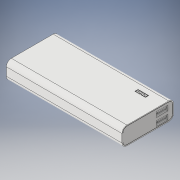
# Autodesk Inventor part: Battery
Saved by Autodesk Inventor 2018 (Build 220112000, 112)
## iProperties
Created: 2018-05-02
Part Number: Battery
Material: Generic
Document SubType Name: Modeling
Designer: Ajith Thomas
Density: 1 g/cm^3
Appearance: Default
Author: Ajith Thomas
Autodesk Inventor part; units mm, degrees
ref_plane "YZ Plane" through (0, 0, 0) normal (1, 0, 0) x (0, 1, 0)
ref_plane "XZ Plane" through (0, 0, 0) normal (0, 1, 0) x (-1, 0, 0)
ref_plane "XY Plane" through (0, 0, 0) normal (0, 0, 1) x (1, 0, 0)
sketch "Sketch1" plane through (0, 0, 0) normal (1, 0, 0) x (0, 1, 0)
  line L0 (11, 31.5) -> (-11, 31.5)
  line L1 (-11, 31.5) -> (-11, -31.5)
  line L2 (-11, -31.5) -> (11, -31.5)
  line L3 (11, -31.5) -> (11, 31.5)
  line L4 (11, 31.5) -> (-11, -31.5) construction
  line L5 (-11, 31.5) -> (11, -31.5) construction
  point P0 (0, 0)
  dimension "d0" = 22
  dimension "d1" = 63
  constraints: 12 end point, 2 midpoint, 2 parallel, 1 horizontal, 1 perpendicular
  measures "d0" distance of L2.end L1.end
  measures "d1" distance of L1.end L0.end
extrude "Extrusion1" add sketch "Sketch1" along normal mid plane 141
fillet "Fillet1" radius 6 4 edges at (0, 11, 31.5) (0, 11, -31.5) (0, -11, 31.5) (0, -11, -31.5)
sketch "Sketch2" plane through (70.5, 0, 0) normal (1, 0, 0) x (0, 0, -1)
  line L0 (10.5, 7) -> (24.5, 7)
  line L1 (24.5, 7) -> (24.5, 1)
  line L2 (24.5, 1) -> (10.5, 1)
  line L3 (10.5, 1) -> (10.5, 7)
  line L4 (31.5, -5) -> (31.5, 5) projected
  line L5 (25.5, 11) -> (-25.5, 11) projected
  line L6 (11.7, 5.85) -> (23.3, 5.85)
  line L7 (23.3, 5.85) -> (23.3, 4.6)
  line L8 (23.3, 4.6) -> (11.7, 4.6)
  line L9 (11.7, 4.6) -> (11.7, 5.85)
  line L10 (10.5, -2.5) -> (24.5, -2.5)
  line L11 (24.5, -2.5) -> (24.5, -8.5)
  line L12 (24.5, -8.5) -> (10.5, -8.5)
  line L13 (10.5, -8.5) -> (10.5, -2.5)
  line L14 (11.7, -3.65) -> (23.3, -3.65)
  line L15 (23.3, -3.65) -> (23.3, -4.9)
  line L16 (23.3, -4.9) -> (11.7, -4.9)
  line L17 (11.7, -4.9) -> (11.7, -3.65)
  point P0 (0, 0)
  dimension "d5" = 14
  dimension "d6" = 6
  dimension "d7" = 7
  dimension "d8" = 4
  dimension "d12" = 1.2
  dimension "d13" = 1.2
  dimension "d14" = 1.15
  dimension "d15" = 3.6
  dimension "d16" = 14
  dimension "d17" = 6
  dimension "d18" = 1.2
  dimension "d19" = 1.2
  dimension "d20" = 1.15
  dimension "d21" = 3.6
  dimension "d22" = 3.5
  constraints: 32 end point, 8 parallel, 4 horizontal, 4 perpendicular
  measures "d5" distance of L1.end L2.end
  measures "d6" distance of L0.end L1.end
  measures "d7" distance between parallel lines of L4 L1
  measures "d8" distance between parallel lines of L5 L0
  measures "d12" distance between parallel lines of L3 L9
  measures "d13" distance between parallel lines of L1 L7
  measures "d14" distance between parallel lines of L0 L6
  measures "d15" distance between parallel lines of L2 L8
  measures "d16" distance of L11.end L12.end
  measures "d17" distance of L10.end L11.end
  measures "d18" distance between parallel lines of L13 L17
  measures "d19" distance between parallel lines of L11 L15
  measures "d20" distance between parallel lines of L10 L14
  measures "d21" distance between parallel lines of L12 L16
  measures "d22" distance between parallel lines of L2 L10
extrude "Extrusion2" cut sketch "Sketch2" against normal blind 10
sketch "Sketch3" plane through (-70.5, 11, -25.5) normal (0, 1, 0) x (1, 0, 0)
  line L0 (110.1613, -6.5149) -> (123.1613, -6.5149)
  line L1 (123.1613, -6.5149) -> (123.1613, -10.5149)
  line L2 (123.1613, -10.5149) -> (110.1613, -10.5149)
  line L3 (110.1613, -10.5149) -> (110.1613, -6.5149)
  line L4 (110.6613, -7.0149) -> (112.6613, -7.0149)
  line L5 (112.6613, -7.0149) -> (112.6613, -10.0149)
  line L6 (112.6613, -10.0149) -> (110.6613, -10.0149)
  line L7 (110.6613, -10.0149) -> (110.6613, -7.0149)
  line L8 (115.9613, -10.0149) -> (113.9613, -10.0149)
  line L9 (113.9613, -10.0149) -> (113.9613, -7.0149)
  line L10 (113.9613, -7.0149) -> (115.9613, -7.0149)
  line L11 (115.9613, -7.0149) -> (115.9613, -10.0149)
  line L12 (119.2613, -10.0149) -> (117.2613, -10.0149)
  line L13 (117.2613, -10.0149) -> (117.2613, -7.0149)
  line L14 (117.2613, -7.0149) -> (119.2613, -7.0149)
  line L15 (119.2613, -7.0149) -> (119.2613, -10.0149)
  line L16 (122.5613, -10.0149) -> (120.5613, -10.0149)
  line L17 (120.5613, -10.0149) -> (120.5613, -7.0149)
  line L18 (120.5613, -7.0149) -> (122.5613, -7.0149)
  line L19 (122.5613, -7.0149) -> (122.5613, -10.0149)
  point P0 (70.5, -25.5)
  dimension "d25" = 13
  dimension "d26" = 4
  dimension "d27" = 2
  dimension "d28" = 3
  dimension "d29" = 0.5
  dimension "d30" = 0.5
  dimension "d33" = 3.3
  constraints: 40 end point, 4 parallel, 3 horizontal, 2 perpendicular, 24 other
  measures "d25" distance of L1.end L2.end
  measures "d26" distance of L0.end L1.end
  measures "d27" distance of L5.end L6.end
  measures "d28" distance of L4.end L5.end
  measures "d29" distance between parallel lines of L0 L4
  measures "d30" distance between parallel lines of L3 L7
  measures "d33" distance of L5.end L8.start
extrude "Extrusion3" cut sketch "Sketch3" against normal blind 0.25
sketch "Sketch4" plane through (70.5, -5, -31.5) normal (0, 0, -1) x (-1, 0, 0)
  line L0 (141, 10) -> (0, 10) construction
  line L1 (0, 0) -> (0, 10) construction
  line L2 (35, 5) -> (42, 5)
  line L3 (42, 5) -> (42, 8)
  line L4 (42, 8) -> (35, 8)
  line L5 (35, 8) -> (35, 5)
  line L6 (38.5, 5) -> (38.5, 8) construction
  line L7 (35, 6.5) -> (36.7876, 5)
  line L8 (35, 6.5) -> (37.3336, 6.5) construction
  line L9 (42, 6.5) -> (40.2124, 5)
  line L10 (42, 6.5) -> (42, 5)
  line L11 (40.2124, 5) -> (42, 5)
  point P0 (70.5, 5)
  dimension "d42" = 3
  dimension "d43" = 35
  dimension "d44" = 7
  dimension "d45" = 2
  dimension "d46" = 40
  constraints: 20 end point, 3 midpoint, 2 horizontal, 2 parallel, 2 perpendicular, 2 symmetric about line, 1 collinear, 1 equal length, 1 point on line
  measures "d42" distance of L3.end L2.end
  measures "d43" distance between parallel lines of L1 L5
  measures "d44" distance between parallel lines of L5 L3
  measures "d45" distance between parallel lines of L0 L4
  measures "d46" angle of L7 L8
extrude "Extrusion4" cut sketch "Sketch4" against normal blind 5 contours L7 L5 L4 L3 L9 L2
sketch "Sketch5" plane through (70.5, -5, -31.5) normal (0, 0, -1) x (-1, 0, 0)
  line L0 (0, 0) -> (0, 10) construction
  line L1 (0, 5) -> (141, 5) construction
  line L2 (141, 10) -> (141, 0) construction
  line L3 (13, 9) -> (27, 9)
  line L4 (27, 9) -> (27, 1)
  line L5 (27, 1) -> (13, 1)
  line L6 (13, 1) -> (13, 9)
  line L7 (13, 9) -> (27, 1) construction
  line L8 (27, 9) -> (13, 1) construction
  line L9 (26.75, 8.75) -> (13.25, 8.75)
  line L10 (13.25, 8.75) -> (13.25, 1.25)
  line L11 (13.25, 1.25) -> (26.75, 1.25)
  line L12 (26.75, 1.25) -> (26.75, 8.75)
  line L13 (35, 6.5) -> (35, 8) projected
  point P0 (70.5, 5)
  point P1 (20, 5)
  dimension "d49" = 14
  dimension "d50" = 8
  dimension "d51" = 0.25
  dimension "d52" = 8
  constraints: 22 end point, 4 midpoint, 4 parallel, 2 perpendicular, 1 horizontal, 1 point on line, 3 other
  measures "d49" distance of L4.end L5.end
  measures "d50" distance of L3.end L4.end
  measures "d51" distance between parallel lines of L3 L9
  measures "d52" distance between parallel lines of L13 L4
extrude "Extrusion5" cut sketch "Sketch5" against normal blind 0.1
sketch "Sketch6" plane through (70.5, 0, 0) normal (1, 0, 0) x (0, 0, -1)
  line L0 (10.5, 1) -> (10.5, 7) projected
  line L1 (10.5, 7) -> (24.5, 7) projected
  line L2 (24.5, 7) -> (24.5, 1) projected
  line L3 (24.5, 1) -> (10.5, 1) projected
  line L4 (10.5, -8.5) -> (10.5, -2.5) projected
  line L5 (10.5, -2.5) -> (24.5, -2.5) projected
  line L6 (24.5, -2.5) -> (24.5, -8.5) projected
  line L7 (24.5, -8.5) -> (10.5, -8.5) projected
  arc A0 (25.5, -11) -> (31.5, -5) centre (25.5, -5) ccw projected
  line L8 (31.5, -5) -> (31.5, 5) projected
  arc A1 (31.5, 5) -> (25.5, 11) centre (25.5, 5) ccw projected
  line L9 (25.5, 11) -> (-25.5, 11) projected
  arc A2 (-25.5, 11) -> (-31.5, 5) centre (-25.5, 5) ccw projected
  line L10 (-31.5, 5) -> (-31.5, -5) projected
  arc A3 (-31.5, -5) -> (-25.5, -11) centre (-25.5, -5) ccw projected
  line L11 (-25.5, -11) -> (25.5, -11) projected
  line L12 (-25.5, 10) -> (25.5, 10)
  arc A4 (30.5, 5) -> (25.5, 10) centre (25.5, 5) ccw
  line L13 (30.5, 5) -> (30.5, -5)
  arc A5 (25.5, -10) -> (30.5, -5) centre (25.5, -5) ccw
  line L14 (25.5, -10) -> (-25.5, -10)
  arc A6 (-30.5, -5) -> (-25.5, -10) centre (-25.5, -5) ccw
  line L15 (-30.5, -5) -> (-30.5, 5)
  arc A7 (-25.5, 10) -> (-30.5, 5) centre (-25.5, 5) ccw
  line L16 (-25.5, 9.75) -> (25.5, 9.75)
  arc A8 (30.25, 5) -> (25.5, 9.75) centre (25.5, 5) ccw
  line L17 (30.25, 5) -> (30.25, -5)
  arc A9 (25.5, -9.75) -> (30.25, -5) centre (25.5, -5) ccw
  line L18 (25.5, -9.75) -> (-25.5, -9.75)
  arc A10 (-30.25, -5) -> (-25.5, -9.75) centre (-25.5, -5) ccw
  line L19 (-30.25, -5) -> (-30.25, 5)
  arc A11 (-25.5, 9.75) -> (-30.25, 5) centre (-25.5, 5) ccw
  point P0 (0, 0)
  dimension "d55" = 1
  dimension "d56" = 1.25
  constraints: 16 end point, 16 point on circle, 8 centre point, 14 other
  measures "d55" distance between parallel lines of L9 L12
  measures "d56" distance between parallel lines of L9 L16
extrude "Extrusion6" cut sketch "Sketch6" against normal blind 0.1 contours L12 A4 L13 A5 L14 A6 L15 A7
mirror "Mirror1" about plane through (0, 0, 0) normal (1, 0, 0) of "Extrusion6"
body "Solid1"
